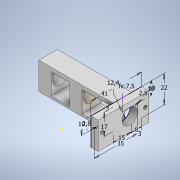
# Autodesk Inventor part: AdaptadorSensorInductivoV2
Saved by Autodesk Inventor 2020.3 (Build 243373000, 373)
## iProperties
Created: 2020-09-07
Part Number: AdaptadorSensorInductivoV2
Material: Generic
Document SubType Name: Modeling
Designer: mifer
Density: 1 g/cm^3
Appearance: Default
Author: mifer
## iProperties of the stored document _3DPrint.ipt
Created: 2020-09-09
Part Number: _3DPrint
Material: Generic
Document SubType Name: Modeling
Designer: mifer
Density: 1 g/cm^3
Appearance: Default
Author: mifer
Autodesk Inventor part; units mm, degrees
ref_plane "YZ Plane" through (0, 0, 0) normal (1, 0, 0) x (0, 1, 0)
ref_plane "XZ Plane" through (0, 0, 0) normal (0, 1, 0) x (-1, 0, 0)
ref_plane "XY Plane" through (0, 0, 0) normal (0, 0, 1) x (1, 0, 0)
sketch "Sketch1" plane through (0, 0, 0) normal (1, 0, 0) x (0, 1, 0)
  line L0 (0, 0) -> (22, 0)
  line L1 (22, 0) -> (22, -41)
  line L2 (22, -41) -> (0, -41)
  line L3 (0, -41) -> (0, 0)
  line L4 (0, -22) -> (0, -32)
  line L5 (22, -33) -> (22, -23)
  circle A0 centre (12, -25.5) radius 6.2
  line L6 (22, -18) -> (0, -18)
  line L7 (0, -18) -> (0, -33)
  line L8 (0, -33) -> (22, -33)
  line L9 (22, -33) -> (22, -18)
  circle A1 centre (12, -3) radius 1.4
  circle A2 centre (12, -38) radius 1.4
  line L10 (19, -18) -> (2, -18)
  line L11 (2, -18) -> (2, -33)
  line L12 (2, -33) -> (19, -33)
  line L13 (19, -33) -> (19, -18)
  point P0 (0, -18)
  dimension "d10" = 41
  dimension "d11" = 22
  dimension "d12" = 15
  dimension "d15" = 10
  dimension "d17" = 8
  dimension "d18" = 2.8
  dimension "d19" = 2.8
  dimension "d20" = 12.4
  dimension "d22" = 10
  dimension "d23" = 10
  dimension "d24" = 35
  dimension "d25" = 3
  dimension "d26" = 7.5
  dimension "d27" = 17
  dimension "d28" = 3
  constraints: 28 end point, 7 parallel, 6 point on line, 3 centre point, 3 horizontal, 3 perpendicular
  measures "d10" distance of L0.end L1.end
  measures "d11" distance of L1.end L2.end
  measures "d12" distance between parallel lines of L8 L6
  measures "d15" distance from line of L1 A0.centre
  measures "d17" distance between parallel lines of L2 L8
  measures "d18" diameter of A1
  measures "d19" diameter of A2
  measures "d20" diameter of A0
  measures "d22" distance from line of L1 A2.centre
  measures "d23" distance from line of L1 A1.centre
  measures "d24" distance of A2.centre A1.centre
  measures "d25" distance from line of L2 A2.centre
  measures "d26" distance from line of L8 A0.centre
  measures "d27" distance between parallel lines of L11 L13
  measures "d28" distance between parallel lines of L13 L9
extrude "Extrusion5" add sketch "Sketch1" along normal blind 6
extrude "Extrusion6" add sketch "Sketch1" against normal blind 50 contours L6 L11 L8 L3 | L1 L8 L13 L6
sketch "Sketch4" plane through (-50, 0, 0) normal (-1, 0, 0) x (0, 0, 1)
  line L0 (-41, 22) -> (-33, 22) projected
  line L1 (-33, 22) -> (-18, 22)
  line L2 (-18, 22) -> (-18, 0)
  line L3 (-18, 0) -> (-33, 0)
  line L4 (-33, 0) -> (-33, 22)
  circle A0 centre (-25.5, 12) radius 6.2 projected
  circle A1 centre (-25.5, 12) radius 6.2
  point P0 (0, 0)
  dimension "d38" = 12.4
  constraints: 8 end point, 2 parallel, 1 centre point, 1 coincident, 1 horizontal, 1 perpendicular
  measures "d38" diameter of A1
extrude "Extrusion7" add sketch "Sketch4" along normal blind 10
ref_plane "Work Plane1" through (-25, 0, 0) normal (1, 0, 0) x (0, 0, -1)
sketch "Sketch5" plane through (-25, 0, 0) normal (1, 0, 0) x (0, 0, -1)
  point P0 (0, 0)
sketch "Sketch6" plane through (-25, 0, 0) normal (1, 0, 0) x (0, 0, -1)
  circle A0 centre (25.5, 12) radius 6.2 projected
  circle A1 centre (25.5, 12) radius 6.2
  line L0 (18, 2) -> (18, 19) projected
  line L1 (33, 0) -> (33, 2) projected
  line L2 (18, 19) -> (33, 19)
  line L3 (33, 19) -> (33, 2)
  line L4 (33, 2) -> (18, 2)
  line L5 (18, 2) -> (18, 19)
  point P0 (0, 0)
  point P1 (18, 2)
  dimension "d39" = 12.4
  constraints: 8 end point, 2 parallel, 1 centre point, 1 coincident, 1 horizontal, 1 perpendicular
  measures "d39" diameter of A1
extrude "Extrusion8" add sketch "Sketch6" against normal blind 10
equation "\"d26\" = 0.5 * d12"
body "Solid2"
